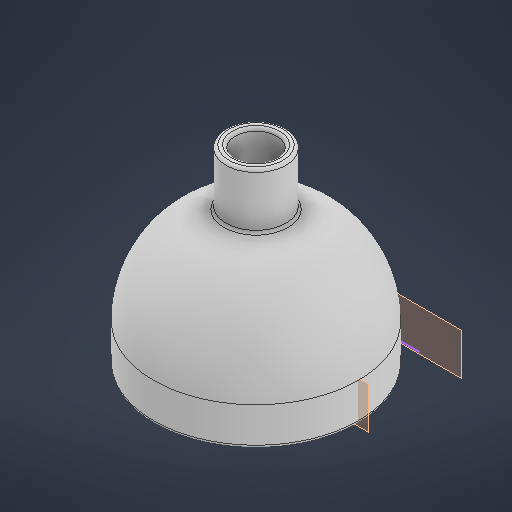
# Autodesk Inventor part: tapag
Saved by Autodesk Inventor 2026.1 (Build 301233020, 233B)
## iProperties
Created: 2025-12-13
Part Number: tapag
Material: Genérico
Document SubType Name: Modeling
Designer: anama
Density: 1 g/cm^3
Appearance: Valor por defecto
Author: anama
Autodesk Inventor part; units mm, degrees
ref_plane "YZ Plane" through (0, 0, 0) normal (1, 0, 0) x (0, 1, 0)
ref_plane "XZ Plane" through (0, 0, 0) normal (0, 1, 0) x (-1, 0, 0)
ref_plane "XY Plane" through (0, 0, 0) normal (0, 0, 1) x (1, 0, 0)
sketch "Boceto1" plane through (0, 0, 0) normal (0, 1, 0) x (-1, 0, 0)
  circle A0 centre (0, 0) radius 40.5
  circle A1 centre (0, 0) radius 44.5
  dimension "d0" = 81
  dimension "d1" = 89
  constraints: 2 centre point, 2 coincident
  measures "d0" diameter of A0
  measures "d1" diameter of A1
extrude "Extrusión1" add sketch "Boceto1" along normal blind 16.5
sketch "Boceto2" plane through (0, 0, 0) normal (0, -1, 0) x (1, 0, 0)
  circle A0 centre (0, 0) radius 40.5 projected
  line L0 (-40.5, 0) -> (40.5, 0)
  line L1 (0, -40.5) -> (-35.4834, -40.5)
  line L2 (-35.4834, -40.5) -> (30.4892, -40.5)
  constraints: 6 end point, 3 point on circle, 2 horizontal, 1 point on line
ref_plane "Plano de trabajo2" through (-35.4834, 0, 0) normal (0, 0, 1) x (1, 0, 0)
ref_plane "Plano de trabajo1" through (-35.4834, 0, -40.5) normal (0, 0, 1) x (1, 0, 0)
sketch "Boceto3" plane through (-35.4834, 0, 0) normal (0, 0, 1) x (1, 0, 0)
  line L0 (79.9834, 0) -> (-9.0166, 0) projected
  line L1 (-9.0166, 0) -> (79.9834, 0)
  line L2 (79.9834, 0) -> (35.4834, 0)
  line L3 (35.4834, 0) -> (35.4834, 16.5)
  line L4 (79.9834, 16.5) -> (-9.0166, 16.5) projected
  circle A0 centre (35.4834, 16.5) radius 44.5
  circle A1 centre (35.4834, 16.5) radius 40.5
  line L5 (35.4834, 57) -> (45.3084, 57)
  line L6 (48.4834, 57) -> (48.4834, 63.6172)
  line L7 (43.2134, 59.0588) -> (27.7534, 59.0588)
  line L8 (35.4834, 57) -> (25.6584, 57)
  line L9 (48.4834, 53.825) -> (48.4834, 54.8569)
  line L10 (22.4834, 53.825) -> (22.4834, 54.8569)
  arc A2 (48.4834, 53.825) -> (45.3084, 57) centre (45.3084, 53.825) ccw
  arc A3 (25.6584, 57) -> (22.4834, 53.825) centre (25.6584, 53.825) ccw
  line L11 (48.4834, 59.0588) -> (44.4834, 59.0588)
  line L12 (22.4834, 59.0588) -> (26.4834, 59.0588)
  line L13 (26.4834, 60.3288) -> (26.4834, 81.7888)
  line L14 (44.4834, 60.3288) -> (44.4834, 81.7888)
  line L15 (48.4834, 59.0588) -> (48.4834, 81.7888)
  line L16 (47.2134, 83.0588) -> (45.7534, 83.0588)
  line L17 (22.4834, 59.0588) -> (22.4834, 81.7888)
  line L18 (23.7534, 83.0588) -> (25.2134, 83.0588)
  arc A4 (45.7534, 83.0588) -> (44.4834, 81.7888) centre (45.7534, 81.7888) ccw
  arc A5 (48.4834, 81.7888) -> (47.2134, 83.0588) centre (47.2134, 81.7888) ccw
  arc A6 (26.4834, 81.7888) -> (25.2134, 83.0588) centre (25.2134, 81.7888) ccw
  arc A7 (23.7534, 83.0588) -> (22.4834, 81.7888) centre (23.7534, 81.7888) ccw
  arc A8 (43.2134, 59.0588) -> (44.4834, 60.3288) centre (43.2134, 60.3288) ccw
  arc A9 (26.4834, 60.3288) -> (27.7534, 59.0588) centre (27.7534, 60.3288) ccw
  line L19 (35.4834, 16.5) -> (35.4834, 85.6826)
  arc A10 (35.4834, 16.5) -> (73.8109, 17.3576) centre (35.4834, 873.3497) ccw
  line L20 (79.9834, 16.5) -> (35.4834, 16.5)
  line L21 (79.9834, 16.5) -> (35.4834, 16.5)
  point P0 (26.4834, 83.0588)
  point P1 (44.4834, 83.0588)
  point P2 (35.4834, 59.0588)
  point P3 (48.2877, 54.9227)
  point P4 (75.9834, 16.5)
  dimension "d5" = 89
  dimension "d6" = 44.5
  dimension "d7" = 89
  dimension "d8" = 81
  dimension "d9" = 13
  dimension "d10" = 26
  dimension "d11" = 3.175
  dimension "d12" = 3.175
  dimension "d13" = 4
  dimension "d14" = 4
  dimension "d15" = 24
  dimension "d16" = 24
  dimension "d17" = 1.27
  dimension "d18" = 1.27
  dimension "d19" = 1.27
  dimension "d20" = 1.27
  dimension "d21" = 1.27
  constraints: 40 end point, 23 point on circle, 19 tangent, 14 point on line, 11 centre point, 5 vertical, 4 perpendicular, 3 collinear, 2 coincident, 2 horizontal, 2 midpoint, 1 equal radius, 1 parallel
  measures "d5" distance of L0.end L0.start
  measures "d6" distance of L0.start L2.end
  measures "d7" diameter of A0
  measures "d8" diameter of A1
  measures "d9" distance of L5.start L6.start
  measures "d10" distance of L11.start L12.start
  measures "d11" radius of A2
  measures "d12" radius of A3
  measures "d13" distance of L11.start L11.end
  measures "d14" distance of L12.start L12.end
  measures "d15" distance of L12.end point (26.483, 83.059)
  measures "d16" distance of L11.end point (44.483, 83.059)
  measures "d17" radius of A4
  measures "d18" radius of A5
  measures "d19" radius of A6
  measures "d20" radius of A7
  measures "d21" radius of A8
revolve "Revolución1" add sketch "Boceto3" angle 360 about axis through (0, 16.5, 0) along (0, 1, 0) contours L4 A1 A2 L5 L19 L7 A8 A0 | A0 A8 L14 A4 L16 A5 L15 L6
fillet "Empalme1" radius 1.27 3 edges at (44.5, 0, 0) (40.5, 0, 0) (-13, 59.0588, 0)
sketch "Boceto4" plane through (0, 59.0588, 0) normal (0, 1, 0) x (1, 0, 0)
  line L0 (0, 0) -> (-5, 0)
  line L1 (0, 0) -> (0, -5)
  line L2 (0, 0) -> (5, 0)
  line L3 (0, 0) -> (0, 5)
  line L4 (5, 0) -> (0, 5)
  line L5 (0, 5) -> (-5, 0)
  line L6 (0, -5) -> (5, 0)
  line L7 (0, -5) -> (-5, 0)
  line L8 (0, 0) -> (-2.5, -2.5)
  line L9 (2.5, 2.5) -> (0, 0)
  line L10 (0, 0) -> (2.5, -2.5)
  line L11 (0, 0) -> (-2.5, 2.5)
  circle A0 centre (-5, 0) radius 1.5
  circle A1 centre (0, -5) radius 1.5
  circle A2 centre (-2.5, -2.5) radius 1
  circle A3 centre (2.5, -2.5) radius 1
  circle A4 centre (5, 0) radius 1.5
  circle A5 centre (2.5, 2.5) radius 1
  circle A6 centre (0, 5) radius 1.5
  circle A7 centre (-2.5, 2.5) radius 1
  circle A8 centre (0, 0) radius 1.5
  dimension "d24" = 5
  dimension "d25" = 5
  dimension "d26" = 5
  dimension "d27" = 5
  dimension "d28" = 3
  dimension "d29" = 3
  dimension "d30" = 2
  dimension "d31" = 2
  dimension "d32" = 3
  dimension "d33" = 2
  dimension "d34" = 3
  dimension "d35" = 2
  dimension "d38" = 3
  constraints: 24 end point, 9 centre point, 9 coincident, 4 midpoint, 2 horizontal, 2 vertical, 1 perpendicular, 1 point on line
  measures "d24" distance of L0.start L0.end
  measures "d25" distance of L0.start L1.end
  measures "d26" distance of L0.start L2.end
  measures "d27" distance of L0.start L3.end
  measures "d28" diameter of A0
  measures "d29" diameter of A1
  measures "d30" diameter of A2
  measures "d31" diameter of A3
  measures "d32" diameter of A4
  measures "d33" diameter of A5
  measures "d34" diameter of A6
  measures "d35" diameter of A7
  measures "d38" diameter of A8
extrude "Extrusión2" cut sketch "Boceto4" against normal blind 3 contours A0 L7 L0 | L0 L5 A0 | L7 A0 L5 | A8 L11 L0 | L0 L8 A8 | L10 A8 L1 | L9 A8 L2 | L11 A8 L3 | L1 A8 L8 | L3 A8 L9 | L2 A8 L10 | A7 L5 | L5 L11 A7 | A2 L8 L7 | L7 A2 | L11 L5 A7 | A2 L7 L8 | A1 L6 L1 | L1 L7 A1 | A4 L4 L2 | L2 L6 A4 | A6 L5 L3 | L3 L4 A6 | A5 L4 L9 | L9 L4 A5 | A3 L6 L10 | L10 L6 A3 | A6 L4 L5 | L7 L6 A1 | L4 A4 L6 | L4 A5 | L6 A3
equation "\"d36\" = d32"
